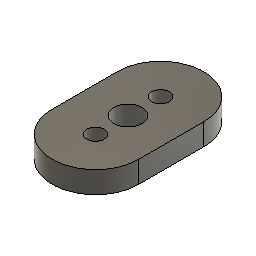
Rod Holder (Autodesk Fusion 360 design; units mm, degrees)
Autodesk Fusion 360 part; units mm, degrees
sketch "Eskiz1" plane through (0, 0, 0) normal (0, 1, 0) x (1, 0, 0)
  circle A0 centre (0, 0) radius 6.5
  circle A1 centre (0, 15) radius 4
  circle A2 centre (0, -15) radius 4
  circle A3 centre (0, 15) radius 20
  circle A4 centre (0, -15) radius 20
  line L0 (-20, 15) -> (-20, -15)
  line L1 (20, 15) -> (20, -15)
  dimension "d1" = 13
  dimension "d2" = 8
  dimension "d3" = 8
  dimension "d4" = 15
  dimension "d5" = 15
  dimension "d6" = 40
  dimension "d7" = 40
  constraint coincident A0.centre origin
  constraint concentric A1 A3
  constraint concentric A2 A4
  constraint coincident A3 L0.start
  constraint coincident A4 L0.end
  constraint tangent A4 L0
  constraint vertical L0
  constraint coincident A3 L1.start
  constraint coincident A4 L1.end
  constraint tangent A4 L1
  constraint parallel L0 L1
  measures "d1" diameter of A0
  measures "d2" diameter of A1
  measures "d3" diameter of A2
  measures "d4" distance of A0.centre A1.centre
  measures "d5" distance of A0.centre A2.centre
  measures "d6" diameter of A3
  measures "d7" diameter of A4
extrude "Ekstrüde Et1" add sketch "Eskiz1" along normal blind 10 contours A0 A3 A4 | A0 A3 A4 | A0 A3 A4 | A0 A3 A4 | A3 A4 L1 | A3 A4 L0 picked at (9.7188, 0) picked at (-9.632, 7.9156) picked at (9.632, -7.9156) picked at (-9.7188, 0)
thread "Diş2" [suppressed]
